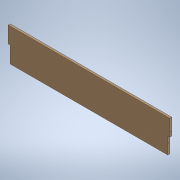
# Autodesk Inventor part: reardraws
Saved by Autodesk Inventor 2022 (Build 260153000, 153)
## iProperties
Created: 2022-02-21
Part Number: reardraws
Material: MDF Medium Density Fiberboard
Document SubType Name: Modeling
Designer: MarkP
Density: 0.8 g/cm^3
Appearance: Cardboard - Corrugated
Author: MarkP
Autodesk Inventor part; units mm, degrees
ref_plane "YZ Plane" through (0, 0, 0) normal (1, 0, 0) x (0, 1, 0)
ref_plane "XZ Plane" through (0, 0, 0) normal (0, 1, 0) x (-1, 0, 0)
ref_plane "XY Plane" through (0, 0, 0) normal (0, 0, 1) x (1, 0, 0)
sketch "Sketch1" plane through (0, 0, 0) normal (0, 0, 1) x (1, 0, 0)
  line L0 (-12, 106.1721) -> (1464, 106.1721)
  line L1 (1464, 106.1721) -> (1464, 406.1721)
  line L2 (1464, 406.1721) -> (-12, 406.1721)
  line L3 (-12, 406.1721) -> (-12, 106.1721)
  line L4 (-12, 406.1721) -> (18, 406.1721)
  line L5 (1464, 406.1721) -> (1446, 406.1721)
  line L6 (1446, 256.1721) -> (1464, 256.1721)
  line L7 (1464, 256.1721) -> (1464, 406.1721)
  line L8 (1446, 256.1721) -> (1446, 106.1721)
  line L9 (-12, 106.1721) -> (6, 106.1721)
  line L10 (6, 106.1721) -> (6, 256.1721)
  line L11 (6, 256.1721) -> (-12, 256.1721)
  line L12 (-12, 256.1721) -> (-12, 106.1721)
  point P0 (0, 0)
  point P1 (18, 106.1721)
  dimension "d1" = 1476
  dimension "d2" = 300
  dimension "d5" = 18
  dimension "d6" = 150
  dimension "d35" = 18
  dimension "d36" = 150
  constraints: 26 end point, 5 parallel, 4 horizontal, 3 perpendicular, 2 point on line
  measures "d1" distance of L2.end L1.end
  measures "d2" distance of L1.end L0.end
  measures "d5" distance of L6.end L6.start
  measures "d6" distance of L6.start L5.end
  measures "d35" distance of L11.end L10.end
  measures "d36" distance of L10.end L9.end
extrude "Extrusion1" add sketch "Sketch1" along normal blind 18 contours L3 L11 L10 L0 | L10 L11 L3 L2 L1 L6 L8 L0
sketch "Sketch2" plane through (-12, 256.1721, 0) normal (-1, 0, 0) x (0, 0, 1)
  line L0 (0, 0) -> (0, 150) projected
  line L1 (0, 150) -> (9, 150)
  line L2 (18, 0) -> (18, 150) projected
  line L3 (0, 150) -> (9, 150) construction
  line L4 (0, 150) -> (18, 150) projected
  line L5 (9, 150) -> (168.25, 150) construction
  line L6 (9, 150) -> (168.25, 150) construction
  line L7 (0, -150) -> (0, 0) projected
  line L8 (9, -9.25) -> (59, -9.25) construction
  circle A0 centre (9, -59.25) radius 2.5
  circle A1 centre (9, 40.75) radius 2.5
  circle A2 centre (9, -9.25) radius 2.5
  point P0 (0, -256.1721)
  dimension "d10" = 0
  dimension "d16" = 159.25
  dimension "d21" = 5
  dimension "d22" = 5
  dimension "d23" = 5
  constraints: 10 end point, 4 horizontal, 3 centre point, 1 coincident, 1 collinear, 1 perpendicular
  measures "d10" distance between parallel lines of L3 L1
  measures "d16" distance of L3.end L8.start
  measures "d21" diameter of A0
  measures "d22" diameter of A1
  measures "d23" diameter of A2
sketch "Sketch3" plane through (1464, 256.1721, 0) normal (1, 0, 0) x (0, 0, -1)
  line L0 (0, 0) -> (0, 150) projected
  line L1 (0, 150) -> (-9, 150)
  circle A0 centre (-9, 40.75) radius 2.5
  circle A1 centre (-9, -9.25) radius 2.5
  circle A2 centre (-9, -59.25) radius 2.5
  point P0 (0, -256.1721)
  dimension "d24" = 9
  dimension "d28" = 5
  dimension "d29" = 5
  dimension "d30" = 5
  constraints: 3 centre point, 2 end point, 1 horizontal
  measures "d24" distance of L0.end L1.end
  measures "d28" diameter of A0
  measures "d29" diameter of A1
  measures "d30" diameter of A2
extrude "Extrusion2" cut sketch "Sketch3" against normal blind 42
extrude "Extrusion3" cut sketch "Sketch2" against normal blind 42
sketch "Sketch4" plane through (0, 0, 0) normal (0, 0, -1) x (-1, 0, 0)
  line L0 (12, 106.1721) -> (-1446, 106.1721) projected
  line L1 (12, 106.1721) -> (-6, 106.1721)
  line L2 (-6, 106.1721) -> (-6, 256.1721)
  line L3 (-6, 256.1721) -> (12, 256.1721)
  line L4 (12, 256.1721) -> (12, 106.1721)
  point P0 (0, 0)
  dimension "d39" = 18
  dimension "d40" = 150
  constraints: 8 end point, 2 parallel, 1 horizontal, 1 perpendicular
  measures "d39" distance of L2.end L3.end
  measures "d40" distance of L1.end L2.end
extrude "Extrusion4" cut sketch "Sketch4" against normal blind 208.825
body "Solid1"
